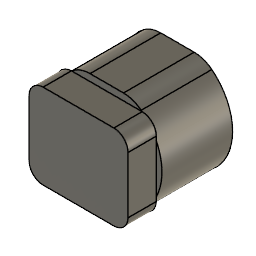
Sleeve (Autodesk Fusion 360 design; units mm, degrees)
Autodesk Fusion 360 part; units mm, degrees
sketch "Sketch1" plane through (0, 0, 0) normal (0, 0, 1) x (1, 0, 0)
  line L0 (0, 0) -> (7, 0)
  line L1 (7, 0) -> (7, 2)
  line L2 (7, 2) -> (0, 2)
  line L3 (0, 2) -> (0, 0)
  dimension "d1" = 7
  dimension "d2" = 2
  constraint horizontal L0
  constraint vertical L1
  constraint horizontal L2
  constraint vertical L3
  constraint coincident L0.start L3.end
  measures "d1" distance of L0.start L0.end
  measures "d2" distance of L0 L2
extrude "Extrude1" add sketch "Sketch1" along normal blind 6
sketch "Sketch2" plane through (0, 2, 0) normal (0, 1, 0) x (-1, 0, 0)
  line L0 (-7, 0) -> (0, 0)
  line L1 (0, 0) -> (0, 6)
  line L2 (0, 6) -> (-7, 6)
  line L3 (-7, 6) -> (-7, 0)
  line L4 (-7, 3) -> (0, 3) construction
  line L5 (-3.5, 6) -> (-3.5, 0) construction
  circle A0 centre (-3.5, 3) radius 2.9
  circle A1 centre (-3.5, 3) radius 3.9
  line L6 (-5.2491, -0.4858) -> (-1.7509, -0.4858)
  line L7 (-5.2491, 6.4858) -> (-1.7509, 6.4858)
  dimension "d5" = 5.8
  dimension "d6" = 1
  constraint midpoint L3 L4.start
  constraint midpoint L1 L4.end
  constraint midpoint L2 L5.start
  constraint midpoint L0 L5.end
  constraint midpoint L5 A0.centre
  constraint coincident A1 L6.start
  constraint coincident A1 L6.end
  constraint horizontal L6
  constraint symmetric L4 L6.start L7.start
  constraint symmetric L4 L6.end L7.end
  measures "d5" diameter of A0
extrude "Extrude2" add sketch "Sketch2" along normal blind 5 contours L0 L1 L2 L3 A1 | L0 A1 L6 | L3 A1 | L1 A1 | L2 A1 L7
fillet "Fillet1" radius 1 4 edges at (0, 1, 6) (0, 1, 0) (7, 1, 0) (7, 1, 6)
fillet "Fillet2" radius 2 4 edges at (1.7509, 4.5, 6.4858) (5.2491, 4.5, 6.4858) (5.2491, 4.5, -0.4858) (1.7509, 4.5, -0.4858)
